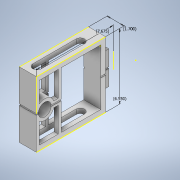
# Autodesk Inventor part: mid side peici
Saved by Autodesk Inventor 2021 (Build 250183000, 183)
## iProperties
Created: 2021-08-21
Part Number: mid side peici
Material: Generic
Document SubType Name: Modeling
Designer: newic
Density: 1 g/cm^3
Appearance: Default
Author: newic
Autodesk Inventor part; units mm, degrees
ref_plane "YZ Plane" through (0, 0, 0) normal (1, 0, 0) x (0, 1, 0)
ref_plane "XZ Plane" through (0, 0, 0) normal (0, 1, 0) x (-1, 0, 0)
ref_plane "XY Plane" through (0, 0, 0) normal (0, 0, 1) x (1, 0, 0)
sketch "Sketch1" plane through (0, 0, 0) normal (0, 1, 0) x (-1, 0, 0)
  line L0 (920.75, 0) -> (0, 0)
  line L1 (0, 0) -> (920.75, 0)
  line L2 (-297.6389, 409.8513) -> (2710.7909, 409.8513) construction
  line L3 (2710.7909, 409.8513) -> (2710.7909, -1716.9746) construction
  line L4 (2710.7909, -1716.9746) -> (-297.6389, -1716.9746) construction
  line L5 (-297.6389, -1716.9746) -> (-297.6389, 409.8513) construction
  line L6 (0, 0) -> (920.75, 0)
  line L7 (920.75, 0) -> (920.75, 100.33)
  line L8 (0, 100.33) -> (920.75, 100.33)
  line L9 (0, 0) -> (0, 100.33)
  line L10 (0, 100.33) -> (0, 120.65)
  line L11 (0, 120.65) -> (920.75, 120.65)
  line L12 (920.75, 120.65) -> (920.75, 100.33)
  line L13 (0, 120.65) -> (0, 196.85)
  line L14 (920.75, 196.85) -> (920.75, 120.65)
  line L15 (477.9962, 0) -> (477.9962, -13.97)
  line L16 (477.9962, -13.97) -> (434.8162, -13.97)
  line L17 (434.8162, -13.97) -> (434.8162, 0)
  line L18 (133.294, 0) -> (133.294, -13.97)
  line L19 (133.294, -13.97) -> (90.114, -13.97)
  line L20 (90.114, -13.97) -> (90.114, 0)
  line L21 (769.0257, 0) -> (769.0257, -13.97)
  line L22 (769.0257, -13.97) -> (812.2057, -13.97)
  line L23 (812.2057, -13.97) -> (812.2057, 0)
  line L24 (434.8162, -13.97) -> (477.9962, -13.97)
  line L25 (769.0257, -13.97) -> (812.2057, -13.97)
  line L26 (90.114, -13.97) -> (133.294, -13.97)
  line L27 (90.114, -13.97) -> (111.704, -13.97)
  line L28 (111.704, -13.97) -> (100.909, -13.97)
  line L29 (100.909, -13.97) -> (122.499, -13.97)
  line L30 (122.499, -13.97) -> (122.499, -33.02)
  line L31 (122.499, -33.02) -> (100.909, -33.02)
  line L32 (100.909, -33.02) -> (100.909, -13.97)
  line L33 (434.8162, -13.97) -> (456.4062, -13.97)
  line L34 (456.4062, -13.97) -> (445.6112, -13.97)
  line L35 (445.6112, -13.97) -> (467.2012, -13.97)
  line L36 (467.2012, -13.97) -> (467.2012, -33.02)
  line L37 (467.2012, -33.02) -> (445.6112, -33.02)
  line L38 (445.6112, -33.02) -> (445.6112, -13.97)
  line L39 (769.0257, -13.97) -> (790.6157, -13.97)
  line L40 (790.6157, -13.97) -> (779.8207, -13.97)
  line L41 (779.8207, -13.97) -> (801.4107, -13.97)
  line L42 (801.4107, -13.97) -> (801.4107, -33.02)
  line L43 (801.4107, -33.02) -> (779.8207, -33.02)
  line L44 (779.8207, -33.02) -> (779.8207, -13.97)
  line L45 (434.8162, 0) -> (413.2262, 0)
  line L46 (413.2262, 0) -> (413.2262, -11.43)
  line L47 (413.2262, -11.43) -> (371.9512, -11.43)
  line L48 (371.9512, -11.43) -> (371.9512, 64.77)
  arc A0 (413.2262, 72.0379) -> (371.9512, 72.0379) centre (392.5887, 68.404) ccw
  line L49 (413.2262, 0) -> (413.2262, 64.77)
  line L50 (371.9512, 64.77) -> (371.9512, 72.0379)
  line L51 (413.2262, 64.77) -> (413.2262, 72.0379)
  line L52 (434.8162, -13.97) -> (434.8162, 202.565)
  line L53 (477.9962, -13.97) -> (477.9962, 202.565)
  line L54 (769.0257, -13.97) -> (769.0257, 202.565)
  line L55 (812.2057, -13.97) -> (812.2057, 202.565)
  line L56 (812.2057, 202.565) -> (769.0257, 202.565)
  line L57 (477.9962, 202.565) -> (434.8162, 202.565)
  line L58 (133.294, -13.97) -> (133.294, 182.245)
  line L59 (90.114, -13.97) -> (90.114, 182.245)
  line L60 (90.114, 182.245) -> (133.294, 182.245)
  line L61 (67.3834, 182.245) -> (164.6776, 182.245)
  line L62 (413.2262, 202.565) -> (508.4774, 202.565)
  line L63 (745.5808, 202.565) -> (847.3717, 202.565)
  line L64 (67.3834, 161.925) -> (164.6776, 161.925)
  line L65 (413.2262, 182.245) -> (508.4774, 182.245)
  line L66 (745.5808, 182.245) -> (847.3717, 182.245)
  line L67 (133.294, -13.97) -> (133.294, 78.74)
  line L68 (133.294, 78.74) -> (434.8162, 78.74)
  line L69 (133.294, -13.97) -> (133.294, 26.67)
  line L70 (133.294, 26.67) -> (371.9512, 26.67)
  line L71 (133.294, 26.67) -> (298.394, 26.67)
  line L72 (298.394, 26.67) -> (317.7759, 78.74)
  line L73 (133.294, 78.74) -> (133.294, 59.055)
  line L74 (133.294, 59.055) -> (310.4486, 59.055)
  point P0 (133.294, 161.925)
  point P1 (90.114, 161.925)
  dimension "d0" = 920.75
  dimension "d1" = 20.32
  dimension "d2" = 76.2
  dimension "d3" = 13.97
  dimension "d4" = 43.18
  dimension "d5" = 13.97
  dimension "d6" = 43.18
  dimension "d7" = 13.97
  dimension "d8" = 13.97
  dimension "d9" = 43.18
  dimension "d10" = 21.59
  dimension "d11" = 19.05
  dimension "d12" = 21.59
  dimension "d13" = 19.05
  dimension "d14" = 21.59
  dimension "d15" = 19.05
  dimension "d16" = 21.59
  dimension "d17" = 11.43
  dimension "d18" = 41.275
  dimension "d19" = 76.2
  dimension "d20" = 20.955
  dimension "d21" = 216.535
  dimension "d22" = 216.535
  dimension "d23" = 216.535
  dimension "d24" = 216.535
  dimension "d25" = 196.215
  dimension "d26" = 20.32
  dimension "d27" = 20.32
  dimension "d28" = 20.32
  dimension "d29" = 92.71
  dimension "d30" = 40.64
  dimension "d31" = 165.1
  dimension "d32" = 19.685
  constraints: 140 end point, 14 perpendicular, 12 horizontal, 11 point on line, 11 vertical, 10 equal length, 7 midpoint, 2 point on circle, 1 centre point, 12 other
  measures "d0" distance of L0.start L0.end
  measures "d1" distance of L8.start L10.end
  measures "d2" distance of L10.end L13.end
  measures "d3" distance of L15.start L15.end
  measures "d4" distance of L15.end L16.end
  measures "d5" distance of L18.start L18.end
  measures "d6" distance of L18.end L19.end
  measures "d7" distance of L19.end L20.end
  measures "d8" distance of L21.start L21.end
  measures "d9" distance of L21.end L22.end
  measures "d10" distance of L30.end L31.end
  measures "d11" distance of L29.end L30.end
  measures "d12" distance of L36.end L37.end
  measures "d13" distance of L35.end L36.end
  measures "d14" distance of L42.end L43.end
  measures "d15" distance of L41.end L42.end
  measures "d16" distance of L17.end L45.end
  measures "d17" distance of L45.end L46.end
  measures "d18" distance of L46.end L47.end
  measures "d19" distance of L47.end L48.end
  measures "d20" radius of A0
  measures "d21" distance of L16.end L52.end
  measures "d22" distance of L24.end L53.end
  measures "d23" distance of L21.end L54.end
  measures "d24" distance of L25.end L55.end
  measures "d25" distance of L26.end L58.end
  measures "d26" distance between parallel lines of L61 L64
  measures "d27" distance between parallel lines of L62 L65
  measures "d28" distance between parallel lines of L63 L66
  measures "d29" distance of L26.end L67.end
  measures "d30" distance of L26.end L69.end
  measures "d31" distance of L69.end L71.end
  measures "d32" distance of L67.end L73.end
extrude "Extrusion1" add sketch "Sketch1" along normal blind 13.97 and the other way blind 152.4 contours L58 L0 L59 L8 | L8 L59 L11 L58 | L18 L19 L20 L0 | L11 L59 L64 L58 | L30 L31 L32 L19
sketch "Sketch2" plane through (-90.114, -152.4, -13.97) normal (1, 0, 0) x (0, 0, -1)
  line L0 (0, 0) -> (0, 166.37) projected
  line L1 (-175.895, 166.37) -> (0, 166.37) projected
  line L2 (-175.895, 166.37) -> (-175.895, 0) projected
  line L3 (0, 0) -> (-175.895, 0) projected
  line L4 (-13.97, 152.4) -> (-13.97, 13.97)
  line L5 (-13.97, 13.97) -> (-161.925, 13.97)
  line L6 (-161.925, 13.97) -> (-161.925, 152.4)
  line L7 (-161.925, 152.4) -> (-13.97, 152.4)
  line L8 (-12.065, 12.065) -> (-12.065, 154.305)
  line L9 (-12.065, 154.305) -> (-163.83, 154.305)
  line L10 (-163.83, 154.305) -> (-163.83, 12.065)
  line L11 (-163.83, 12.065) -> (-12.065, 12.065)
  line L12 (-12.065, 70.3973) -> (-112.5728, 70.3973)
  line L13 (-112.5728, 70.3973) -> (-112.5728, 191.5999)
  line L14 (-112.5728, 70.3973) -> (-112.5728, -17.578)
  circle A0 centre (-150.6728, 83.185) radius 38.1
  line L15 (0, 0) -> (19.05, 0) projected
  line L16 (0, 0) -> (0, 83.185)
  line L17 (0, 0) -> (0, 166.37) projected
  line L18 (19.05, 166.37) -> (0, 166.37) projected
  line L19 (0, 166.37) -> (0, 83.185)
  line L20 (0, 124.7775) -> (67.1734, 124.7775)
  line L21 (67.1734, 124.7775) -> (67.1734, 184.1281)
  line L22 (67.1734, 184.1281) -> (0, 184.1281)
  line L23 (0, 184.1281) -> (0, 124.7775)
  line L24 (19.05, 0) -> (19.05, 166.37) projected
  line L25 (19.05, 0) -> (19.05, 83.185)
  line L26 (19.05, 41.5925) -> (0, 41.5925)
  line L27 (0, 41.5925) -> (0, -34.1667)
  line L28 (0, -34.1667) -> (19.05, -34.1667)
  line L29 (19.05, -34.1667) -> (19.05, 41.5925)
  point P0 (-13.97, 152.4)
  point P1 (-112.5728, 12.065)
  point P2 (-112.5728, 154.305)
  dimension "d39" = 13.97
  dimension "d40" = 1.905
  dimension "d41" = 100.5078
  constraints: 44 end point, 5 equal length, 4 midpoint, 3 perpendicular, 2 horizontal, 2 point on line, 2 vertical, 1 centre point, 1 tangent, 6 other
  measures "d39" distance between parallel lines of L0 L4
  measures "d40" distance between parallel lines of L4 L8
  measures "d41" distance of L12.start L12.end
extrude "Extrusion2" cut sketch "Sketch2" against normal through all contours L0 L26 L24 L15 | L15 L29 L28 L27 | L14 L5 L4 L12 L8 L11 | L0 L18 L24 L20 | L14 L12 L4 L5 | L23 L22 L21 L20 L24 L18 | L12 L4 L7 L13 L9 L8 | L13 L7 L4 L12
sketch "Sketch3" plane through (-90.114, -152.4, -13.97) normal (1, 0, 0) x (0, 0, -1)
  line L0 (-196.2151, 166.37) -> (-196.2151, 0)
  line L1 (-12.0651, 154.305) -> (-112.5729, 154.305)
  line L2 (-12.0651, 12.065) -> (-12.0651, 154.305)
  line L3 (-0.0001, 0) -> (-0.0001, 166.37)
  line L4 (-112.5729, 12.065) -> (-12.0651, 12.065)
  line L5 (-0.0001, 166.37) -> (-196.2151, 166.37)
  line L6 (-196.2151, 0) -> (-0.0001, 0)
  line L7 (-112.5729, 154.305) -> (-112.5729, 12.065)
  line L8 (-120.104, 12.065) -> (-120.104, 52.9441)
  circle A0 centre (-154.394, 83.185) radius 38.1
  arc A1 (-188.684, 52.9441) -> (-120.104, 52.9441) centre (-154.394, 83.185) ccw
  line L9 (-188.684, 52.9441) -> (-188.684, 12.065)
  line L10 (-188.684, 12.065) -> (-120.104, 12.065)
  line L11 (-42.5451, 166.37) -> (-42.5451, 154.305)
  line L12 (-120.104, 113.4259) -> (-120.104, 154.4562)
  arc A2 (-120.104, 113.4259) -> (-188.684, 113.4259) centre (-154.394, 83.185) ccw
  line L13 (-188.684, 154.4562) -> (-188.684, 113.4259)
  line L14 (-120.104, 154.4562) -> (-188.684, 154.4562)
  circle A3 centre (-154.394, 83.185) radius 16.3195
  point P0 (-182.2451, 152.4)
  point P1 (-13.9701, 152.4)
  dimension "d46" = 32.639
  constraints: 30 end point, 4 centre point, 4 point on circle
  measures "d46" diameter of A3
extrude "Extrusion3" cut sketch "Sketch3" against normal through all contours A3
sketch "Sketch4" plane through (-90.114, -152.4, -13.97) normal (1, 0, 0) x (0, 0, -1)
  line L0 (-196.2151, 166.37) -> (-196.2151, 0)
  line L1 (-120.104, 113.4259) -> (-120.104, 154.4562)
  line L2 (-120.104, 12.065) -> (-120.104, 52.9441)
  line L3 (-120.104, 154.4562) -> (-188.684, 154.4562)
  line L4 (-188.684, 154.4562) -> (-188.684, 113.4259)
  line L5 (-188.684, 52.9441) -> (-188.684, 12.065)
  line L6 (-188.684, 12.065) -> (-120.104, 12.065)
  line L7 (-12.0651, 154.305) -> (-112.5729, 154.305)
  line L8 (-12.0651, 12.065) -> (-12.0651, 154.305)
  line L9 (-112.5729, 154.305) -> (-112.5729, 12.065)
  line L10 (-0.0001, 166.37) -> (-196.2151, 166.37)
  line L11 (-196.2151, 0) -> (-0.0001, 0)
  line L12 (-112.5729, 12.065) -> (-12.0651, 12.065)
  line L13 (-42.5451, 166.37) -> (-42.5451, 154.305)
  line L14 (-0.0001, 0) -> (-0.0001, 166.37)
  circle A0 centre (-154.394, 83.185) radius 16.3195
  circle A1 centre (-154.394, 83.185) radius 23.9395
  circle A2 centre (-154.394, 83.185) radius 16.3195 projected
  line L15 (-138.0745, 83.185) -> (-107.0212, 83.185)
  line L16 (-138.0745, 90.805) -> (-107.0212, 90.805)
  line L17 (-138.0745, 75.565) -> (-107.0212, 75.565)
  line L18 (-138.0745, 75.565) -> (-139.9627, 75.565)
  line L19 (-138.0745, 90.805) -> (-139.9627, 90.805)
  circle A3 centre (-154.394, 83.185) radius 16.3195 projected
  line L20 (-12.065, 12.065) -> (-112.5728, 12.065) projected
  line L21 (-112.5728, 12.065) -> (-112.5728, 154.305) projected
  line L22 (-112.5728, 154.305) -> (-12.065, 154.305) projected
  line L23 (-12.065, 154.305) -> (-12.065, 12.065) projected
  line L24 (0, 0) -> (0, 166.37) projected
  line L25 (-175.895, 166.37) -> (0, 166.37) projected
  line L26 (-175.895, 166.37) -> (-175.895, 0) projected
  line L27 (0, 0) -> (-175.895, 0) projected
  line L28 (-175.895, -12.7057) -> (-175.895, 174.9983)
  line L29 (-168.275, -12.7057) -> (-168.275, 174.9983)
  line L30 (-120.104, 52.9441) -> (-120.104, 113.4259)
  point P0 (-13.97, 152.4)
  point P1 (-182.2451, 152.4)
  point P2 (-13.9701, 152.4)
  point P3 (-168.275, 154.4562)
  point P4 (-168.275, 102.6893)
  point P5 (-131.6996, 90.805)
  point P6 (-120.104, 90.805)
  point P7 (-120.104, 75.565)
  point P8 (-131.6996, 75.565)
  point P9 (-168.275, 63.6807)
  point P10 (-168.275, 12.065)
  dimension "d49" = 32.639
  dimension "d50" = 47.879
  dimension "d51" = 7.62
  dimension "d52" = 7.62
  dimension "d53" = 7.62
  constraints: 46 end point, 3 horizontal, 3 parallel, 3 point on circle, 2 centre point, 1 coincident, 1 collinear, 1 perpendicular
  measures "d49" diameter of A0
  measures "d50" diameter of A1
  measures "d51" distance between parallel lines of L15 L16
  measures "d52" distance between parallel lines of L15 L17
  measures "d53" distance between parallel lines of L28 L29
extrude "Extrusion4" cut sketch "Sketch4" against normal through all contours L3 L1 L30 L16 A1 L29 | L29 A1 L17 L30 L2 L6
sketch "Sketch5" plane through (0, -152.4, 0) normal (0, -1, 0) x (1, 0, 0)
  line L0 (-90.114, -13.97) -> (-133.294, -13.97) projected
  line L1 (-111.704, -13.97) -> (-111.704, 17.78)
  line L2 (-133.294, 161.925) -> (-90.114, 161.925) projected
  line L3 (-111.704, 161.925) -> (-111.704, 149.225)
  circle A0 centre (-111.704, 28.575) radius 10.795
  circle A1 centre (-111.704, 138.43) radius 10.795
  line L4 (-90.114, -13.97) -> (-90.114, 161.925) projected
  line L5 (-122.499, 143.9608) -> (-122.499, 4.5606)
  line L6 (-100.909, 151.8855) -> (-100.909, 12.2046)
  point P0 (0, 0)
  point P1 (-122.499, 138.43)
  point P2 (-122.499, 28.575)
  point P3 (-100.909, 28.575)
  point P4 (-100.909, 138.43)
  dimension "d0" = 920.75
  dimension "d56" = 31.75
  dimension "d57" = 12.7
  dimension "d60" = 21.59
  dimension "d61" = 42.545
  dimension "d62" = 21.59
  dimension "d63" = 21.59
  dimension "d64" = 21.59
  dimension "d65" = 23.495
  constraints: 8 end point, 3 tangent, 3 vertical, 2 centre point, 2 midpoint
  measures "d56" distance of L1.start L1.end
  measures "d57" distance of L3.start L3.end
  measures "d60" distance from line of L4 A0.centre
  measures "d61" distance from line of L0 A0.centre
  measures "d62" diameter of A0
  measures "d63" diameter of A1
  measures "d64" distance from line of L4 A1.centre
  measures "d65" distance from line of L2 A1.centre
extrude "Extrusion5" cut sketch "Sketch5" against normal through all contours A0 | A0 L5 A1 L6 | A1
sketch "Sketch6" plane through (-90.114, -152.4, -13.97) normal (1, 0, 0) x (0, 0, -1)
  circle A0 centre (-154.394, 83.185) radius 16.3195 projected
  circle A1 centre (-154.394, 83.185) radius 23.9395
  circle A2 centre (-154.394, 83.185) radius 16.3195
  line L0 (-175.895, 166.37) -> (-175.895, 0) projected
  line L1 (-175.895, 72.6586) -> (-175.895, 93.7114)
  point P0 (-13.97, 152.4)
  dimension "d68" = 32.639
  constraints: 2 centre point, 2 coincident, 2 end point, 2 point on circle, 2 point on line
  measures "d68" diameter of A2
extrude "Extrusion6" add sketch "Sketch6" against normal blind 34.29 contours A1 L0 picked at (-174.1678, 83.185)
sketch "Sketch7" plane through (-122.499, -110.8075, -13.97) normal (0, -1, 0) x (1, 0, 0)
  line L0 (21.59, -19.05) -> (0, -19.05) projected
  line L1 (0, -19.05) -> (21.59, -19.05)
  line L2 (21.59, -19.05) -> (21.59, 0)
  line L3 (-10.795, 0) -> (32.385, 0) projected
  circle A0 centre (10.795, -9.525) radius 4.445
  point P0 (122.499, 13.97)
  dimension "d71" = 8.89
  constraints: 4 end point, 1 centre point, 1 collinear, 1 perpendicular, 1 point on line
  measures "d71" diameter of A0
extrude "Extrusion7" cut sketch "Sketch7" against normal through all
sketch "Sketch8" plane through (-133.294, 13.97, 161.925) normal (0, 0, 1) x (1, 0, 0)
  line L0 (32.385, -11.9138) -> (32.385, -75.565) projected
  line L1 (0, -166.37) -> (0, 0) projected
  line L2 (43.18, 0) -> (43.18, -166.37) projected
  line L3 (0, 0) -> (43.18, 0) projected
  line L4 (0, -166.37) -> (0, 0) projected
  line L5 (43.18, -166.37) -> (0, -166.37) projected
  line L6 (0, -154.305) -> (0, -12.065) projected
  line L7 (0, -83.185) -> (85.68, -83.185)
  line L8 (0, -81.28) -> (85.68, -81.28)
  line L9 (0, -85.09) -> (85.68, -85.09)
  point P0 (133.294, -13.97)
  point P1 (43.18, -85.09)
  point P2 (43.18, -81.28)
  dimension "d74" = 1.905
  dimension "d75" = 1.905
  constraints: 6 end point, 2 parallel, 1 horizontal, 1 midpoint
  measures "d74" distance between parallel lines of L7 L8
  measures "d75" distance between parallel lines of L7 L9
extrude "Extrusion8" cut sketch "Sketch8" against normal blind 1.27 contours L1 L7 L2 L9 | L1 L8 L2 L7
sketch "Sketch9" plane through (-90.114, -152.4, -13.97) normal (1, 0, 0) x (0, 0, -1)
  line L0 (-175.895, 81.28) -> (-174.625, 81.28) projected
  line L1 (-175.26, 81.28) -> (-168.3969, 81.28)
  line L2 (-168.3969, 81.28) -> (-168.3969, 85.09)
  line L3 (-168.3969, 85.09) -> (-175.26, 85.09)
  line L4 (-175.26, 85.09) -> (-175.26, 81.28)
  point P0 (-13.97, 152.4)
  constraints: 8 end point, 2 parallel, 1 horizontal, 1 midpoint, 1 perpendicular
extrude "Extrusion9" cut sketch "Sketch9" against normal blind 1.27
sketch "Sketch10" plane through (-133.294, -152.4, -13.97) normal (-1, 0, 0) x (0, 0, 1)
  line L0 (175.895, 81.28) -> (174.625, 81.28) projected
  line L1 (175.26, 81.28) -> (168.0363, 81.28)
  line L2 (168.0363, 81.28) -> (168.0363, 85.09)
  line L3 (168.0363, 85.09) -> (175.26, 85.09)
  line L4 (175.26, 85.09) -> (175.26, 81.28)
  point P0 (13.97, 152.4)
  constraints: 8 end point, 2 parallel, 1 horizontal, 1 midpoint, 1 perpendicular
extrude "Extrusion10" cut sketch "Sketch10" against normal blind 1.27
sketch "Sketch11" plane through (-122.499, -110.8075, -33.02) normal (-1, 0, 0) x (0, 0, 1)
  line L0 (19.05, 83.185) -> (0, 83.185) projected
  line L1 (0, 0) -> (0, 83.185) projected
  line L2 (0, 0) -> (19.05, 0) projected
  line L3 (19.05, 0) -> (19.05, 83.185) projected
  line L4 (0, 0) -> (0, 83.185) projected
  line L5 (0, 41.5925) -> (46.553, 41.5925)
  line L6 (0, 39.6875) -> (46.553, 39.6875)
  line L7 (0, 43.4975) -> (46.553, 43.4975)
  point P0 (33.02, 110.8075)
  point P1 (19.05, 43.4975)
  point P2 (0, 43.4975)
  point P3 (0, 39.6875)
  point P4 (19.05, 39.6875)
  dimension "d82" = 1.905
  dimension "d83" = 1.905
  constraints: 6 end point, 2 parallel, 1 horizontal, 1 midpoint
  measures "d82" distance between parallel lines of L5 L6
  measures "d83" distance between parallel lines of L5 L7
extrude "Extrusion11" cut sketch "Sketch11" against normal blind 1.27 contours L3 L5 L1 L7 | L3 L6 L1 L5
sketch "Sketch12" plane through (-133.294, -152.4, -13.97) normal (-1, 0, 0) x (0, 0, 1)
  line L0 (-19.05, 85.09) -> (0, 85.09) projected
  line L1 (-1.3457, 85.09) -> (16.2492, 85.09)
  line L2 (16.2492, 85.09) -> (16.2492, 81.28)
  line L3 (16.2492, 81.28) -> (-1.3457, 81.28)
  line L4 (-1.3457, 81.28) -> (-1.3457, 85.09)
  point P0 (13.97, 152.4)
  constraints: 8 end point, 2 parallel, 1 horizontal, 1 perpendicular, 1 point on line
extrude "Extrusion12" cut sketch "Sketch12" against normal blind 1.27
sketch "Sketch13" plane through (-90.114, 13.97, -13.97) normal (0, 0, -1) x (-1, 0, 0)
  line L0 (0, -85.09) -> (43.18, -85.09) projected
  line L1 (42.667, -85.09) -> (-4.3743, -85.09)
  line L2 (-4.3743, -85.09) -> (-4.3743, -81.28)
  line L3 (-4.3743, -81.28) -> (42.667, -81.28)
  line L4 (42.667, -81.28) -> (42.667, -85.09)
  line L5 (31.115, -81.28) -> (31.115, -85.09) projected
  line L6 (31.115, -85.09) -> (31.115, -81.28)
  line L7 (10.795, -124.7775) -> (10.795, -41.5925) projected
  line L8 (10.795, -85.09) -> (10.795, -81.28)
  point P0 (-90.114, -13.97)
  constraints: 12 end point, 5 point on line, 3 equal length, 1 horizontal, 1 perpendicular
extrude "Extrusion13" cut sketch "Sketch13" against normal blind 1.27 contours L1 L2 L3 L7 L0 | L5 L3 L4 L0
sketch "Sketch14" plane through (-100.909, -27.6225, -33.02) normal (0, 0, -1) x (-1, 0, 0)
  line L0 (32.385, -43.4975) -> (21.59, -43.4975) projected
  line L1 (32.385, -39.6875) -> (-10.795, -39.6875) projected
  line L2 (21.9999, -43.4975) -> (-3.8997, -43.4975)
  line L3 (-3.8997, -43.4975) -> (-3.8997, -39.6875)
  line L4 (-3.8997, -39.6875) -> (21.9999, -39.6875)
  line L5 (21.9999, -39.6875) -> (21.9999, -43.4975)
  point P0 (-100.909, 27.6225)
  constraints: 8 end point, 2 parallel, 2 point on line, 1 horizontal, 1 perpendicular
extrude "Extrusion14" cut sketch "Sketch14" against normal blind 1.27
sketch "Sketch15" plane through (-100.909, -27.6225, -13.97) normal (1, 0, 0) x (0, 0, -1)
  line L0 (-12.065, -43.4975) -> (0, -43.4975) projected
  line L1 (-0.6678, -43.4975) -> (23.2828, -43.4975)
  line L2 (23.2828, -43.4975) -> (23.2828, -39.6875)
  line L3 (23.2828, -39.6875) -> (-0.6678, -39.6875)
  line L4 (-0.6678, -39.6875) -> (-0.6678, -43.4975)
  line L5 (-1.27, -43.4975) -> (-1.27, -39.6875) projected
  line L6 (19.05, -39.6875) -> (0, -39.6875) projected
  line L7 (-1.27, -43.4975) -> (8.5133, -43.4975)
  line L8 (8.5133, -43.4975) -> (8.5133, -39.6875)
  line L9 (8.5133, -39.6875) -> (-1.27, -39.6875)
  line L10 (-1.27, -39.6875) -> (-1.27, -43.4975)
  point P0 (-13.97, 27.6225)
  constraints: 16 end point, 4 parallel, 2 horizontal, 2 perpendicular, 2 point on line
extrude "Extrusion15" cut sketch "Sketch15" against normal blind 1.27
sketch "Sketch16" plane through (-90.114, 13.97, 161.925) normal (1, 0, 0) x (0, 0, -1)
  line L0 (194.945, -81.28) -> (175.895, -81.28) projected
  line L1 (177.3654, -81.28) -> (158.7871, -81.28)
  line L2 (158.7871, -81.28) -> (158.7871, -85.09)
  line L3 (158.7871, -85.09) -> (177.3654, -85.09)
  line L4 (177.3654, -85.09) -> (177.3654, -81.28)
  point P0 (161.925, -13.97)
  constraints: 8 end point, 2 parallel, 1 horizontal, 1 perpendicular, 1 point on line
extrude "Extrusion16" cut sketch "Sketch16" against normal blind 1.27
sketch "Sketch17" plane through (-133.294, -152.4, -13.97) normal (-1, 0, 0) x (0, 0, 1)
  line L0 (12.065, 85.09) -> (1.27, 85.09) projected
  line L1 (170.6019, 81.28) -> (175.895, 81.28) projected
  line L2 (4.2707, 85.09) -> (173.2485, 85.09)
  line L3 (173.2485, 85.09) -> (173.2485, 81.28)
  line L4 (173.2485, 81.28) -> (4.2707, 81.28)
  line L5 (4.2707, 81.28) -> (4.2707, 85.09)
  line L6 (142.9288, 85.09) -> (98.9205, 85.09)
  line L7 (98.9205, 85.09) -> (98.9205, 81.28)
  line L8 (98.9205, 81.28) -> (142.9288, 81.28)
  line L9 (142.9288, 81.28) -> (142.9288, 85.09)
  point P0 (13.97, 152.4)
  constraints: 16 end point, 4 parallel, 3 point on line, 2 horizontal, 2 perpendicular, 1 midpoint
extrude "Extrusion17" cut sketch "Sketch17" against normal blind 1.27 contours L2 L9 L4 L7
sketch "Sketch18" plane through (-90.114, 13.97, 161.925) normal (1, 0, 0) x (0, 0, -1)
  line L0 (175.895, -81.28) -> (163.83, -81.28) projected
  line L1 (0, -85.09) -> (5.2931, -85.09) projected
  line L2 (169.8625, -81.28) -> (3.2831, -81.28)
  line L3 (3.2831, -81.28) -> (3.2831, -85.09)
  line L4 (3.2831, -85.09) -> (169.8625, -85.09)
  line L5 (169.8625, -85.09) -> (169.8625, -81.28)
  line L6 (27.0349, -85.09) -> (70.2725, -85.09)
  line L7 (70.2725, -85.09) -> (70.2725, -81.28)
  line L8 (70.2725, -81.28) -> (27.0349, -81.28)
  line L9 (27.0349, -81.28) -> (27.0349, -85.09)
  point P0 (161.925, -13.97)
  constraints: 16 end point, 4 parallel, 3 point on line, 2 horizontal, 2 perpendicular, 1 midpoint
extrude "Extrusion18" cut sketch "Sketch18" against normal blind 1.27 contours L7 L4 L9 L2
sketch "Sketch19" plane through (-122.499, 1.905, 98.6028) normal (0, 0, -1) x (-1, 0, 0)
  line L0 (9.525, -69.215) -> (10.795, -69.215) projected
  line L1 (-31.115, -73.025) -> (-32.385, -73.025) projected
  line L2 (10.795, -69.215) -> (-32.385, -69.215)
  line L3 (-32.385, -69.215) -> (-32.385, -73.025)
  line L4 (-32.385, -73.025) -> (10.795, -73.025)
  line L5 (10.795, -73.025) -> (10.795, -69.215)
  point P0 (-122.499, -1.905)
  constraints: 8 end point, 2 parallel, 1 horizontal, 1 perpendicular
extrude "Extrusion19" cut sketch "Sketch19" against normal blind 1.27
sketch "Sketch20" plane through (-100.909, -152.4, 28.575) normal (-1, 0, 0) x (0, 0, 1)
  line L0 (70.0278, 85.09) -> (71.2978, 85.09) projected
  line L1 (71.2978, 85.09) -> (71.2978, 81.28) projected
  line L2 (71.2978, 81.28) -> (70.0278, 81.28) projected
  line L3 (70.0278, 12.065) -> (70.0278, 81.28) projected
  line L4 (0, 12.065) -> (70.0278, 12.065) projected
  line L5 (0, 0) -> (0, 12.065) projected
  line L6 (109.855, 0) -> (0, 0) projected
  line L7 (109.855, 0) -> (109.855, 12.065) projected
  line L8 (77.559, 12.065) -> (109.855, 12.065) projected
  line L9 (77.559, 75.565) -> (77.559, 12.065) projected
  line L10 (89.1546, 75.565) -> (77.559, 75.565) projected
  arc A0 (89.1546, 90.805) -> (89.1546, 75.565) centre (111.849, 83.185) ccw projected
  line L11 (77.559, 90.805) -> (89.1546, 90.805) projected
  line L12 (77.559, 154.4562) -> (77.559, 90.805) projected
  line L13 (109.855, 154.4562) -> (77.559, 154.4562) projected
  line L14 (109.855, 154.4562) -> (109.855, 166.37) projected
  line L15 (0, 166.37) -> (109.855, 166.37) projected
  line L16 (0, 154.305) -> (0, 166.37) projected
  line L17 (70.0278, 154.305) -> (0, 154.305) projected
  line L18 (70.0278, 85.09) -> (70.0278, 154.305) projected
  line L19 (70.0278, 85.09) -> (91.0706, 85.09)
  line L20 (91.0706, 85.09) -> (91.0706, 81.28)
  line L21 (91.0706, 81.28) -> (70.0278, 81.28)
  line L22 (70.0278, 81.28) -> (70.0278, 85.09)
  point P0 (-28.575, 152.4)
  point P1 (87.9854, 81.28)
  point P2 (87.9854, 85.09)
  constraints: 8 end point, 2 parallel, 1 horizontal, 1 perpendicular
extrude "Extrusion20" cut sketch "Sketch20" against normal blind 1.27 contours L19 A0 L21 L1
sketch "Sketch21" plane through (-122.499, -152.4, 138.43) normal (1, 0, 0) x (0, 0, -1)
  line L0 (38.5572, 85.09) -> (39.8272, 85.09) projected
  line L1 (39.8272, 154.305) -> (39.8272, 85.09) projected
  line L2 (109.855, 154.305) -> (39.8272, 154.305) projected
  line L3 (109.855, 154.305) -> (109.855, 166.37) projected
  line L4 (0, 166.37) -> (109.855, 166.37) projected
  line L5 (0, 154.4562) -> (0, 166.37) projected
  line L6 (32.296, 154.4562) -> (0, 154.4562) projected
  line L7 (32.296, 90.805) -> (32.296, 154.4562) projected
  line L8 (20.7004, 90.805) -> (32.296, 90.805) projected
  arc A0 (20.7004, 75.565) -> (20.7004, 90.805) centre (-1.994, 83.185) ccw projected
  line L9 (32.296, 75.565) -> (20.7004, 75.565) projected
  line L10 (32.296, 12.065) -> (32.296, 75.565) projected
  line L11 (0, 12.065) -> (32.296, 12.065) projected
  line L12 (0, 0) -> (0, 12.065) projected
  line L13 (109.855, 0) -> (0, 0) projected
  line L14 (109.855, 0) -> (109.855, 12.065) projected
  line L15 (39.8272, 12.065) -> (109.855, 12.065) projected
  line L16 (39.8272, 81.28) -> (39.8272, 12.065) projected
  line L17 (39.8272, 81.28) -> (38.5572, 81.28) projected
  line L18 (38.5572, 81.28) -> (38.5572, 85.09) projected
  line L19 (39.8272, 81.28) -> (20.7004, 81.28)
  line L20 (20.7004, 81.28) -> (20.7004, 85.09)
  line L21 (20.7004, 85.09) -> (39.8272, 85.09)
  line L22 (39.8272, 85.09) -> (39.8272, 81.28)
  point P0 (138.43, 152.4)
  point P1 (21.8696, 85.09)
  point P2 (21.8696, 81.28)
  constraints: 8 end point, 2 parallel, 1 horizontal, 1 perpendicular
extrude "Extrusion21" cut sketch "Sketch21" against normal blind 1.27 contours L18 L19 A0 L21
sketch "Sketch22" plane through (-90.114, 13.97, 161.925) normal (1, 0, 0) x (0, 0, -1)
  line L0 (194.945, -81.28) -> (194.945, -41.5925) projected
  line L1 (0, 0) -> (0, -81.28) projected
  line L2 (175.895, -166.37) -> (0, -166.37) projected
  line L3 (0, 0) -> (175.895, 0) projected
  point P0 (161.925, -13.97)
  dimension "d106" = 194.945
  dimension "d107" = 166.37
  measures "d106" distance between parallel lines of L0 L1
  measures "d107" distance between parallel lines of L2 L3
sketch "Sketch23" plane through (0, 13.97, 0) normal (0, 1, 0) x (1, 0, 0)
  line L0 (-133.294, 13.97) -> (-133.294, -161.925) projected
  line L1 (-90.114, -161.925) -> (-90.114, 13.97) projected
  point P0 (0, 0)
  dimension "d108" = 43.18
  measures "d108" distance between parallel lines of L0 L1
body "Solid1"
